Autodesk Fusion 360 part; units mm, degrees
(part 6 of 6)
sketch "Sketch1" plane through (0, 0, 0) normal (0, 0, 1) x (1, 0, 0)
  circle A0 centre (0, 0) radius 18.6 construction
  line L0 (-40.1145, 10.4906) -> (-17.9049, -15.3744)
  line L1 (5, 25.3685) -> (5, 26.9321) construction
  line L2 (-5, 26.019) -> (-5, 25.3685)
  line L3 (-5, 40) -> (-36.5447, 26.1628)
  line L4 (-28.8171, 18.6328) -> (-7.8034, 27.8505)
  line L5 (-29.888, 13.9311) -> (-26.2116, 9.6495)
  arc A1 (-36.5447, 26.1628) -> (-40.1145, 10.4906) centre (-32.5276, 17.0051) ccw
  line L6 (15.2, 40) -> (15.2, 36.8) construction
  line L7 (15.2, 36.8) -> (0, 36.8) construction
  line L8 (0, 36.8) -> (0, 40) construction
  line L9 (15.2, 40) -> (55, 40) construction
  line L10 (70.2, 40) -> (70.2, 36.8) construction
  line L11 (70.2, 36.8) -> (55, 36.8) construction
  line L12 (55, 36.8) -> (55, 40) construction
  line L13 (-5, 40) -> (0, 40) construction
  line L14 (41.6, 0) -> (41.6, 20) construction
  arc A2 (90, 30) -> (90, 40) centre (90, 35) ccw construction
  line L15 (90, 30) -> (51.6, 30) construction
  line L16 (8, 29.9321) -> (28.6, 29.9321) construction
  line L17 (31.6, 26.9321) -> (31.6, 12.775) construction
  arc A3 (-17.9049, -15.3744) -> (-13.0046, -19.6936) centre (0, 0) ccw
  arc A4 (21.5214, 9.6845) -> (7.0977, 22.5074) centre (0, 0) ccw construction
  arc A5 (-7.0977, 22.5074) -> (-21.236, 10.2952) centre (0, 0) ccw
  arc A6 (22.9714, -5.4105) -> (41.6, 0) centre (31.5, 0) ccw construction
  arc A7 (29.2641, 9.8494) -> (25.9158, 8.4159) centre (31.5, 0) ccw construction
  arc A8 (-28.8171, 18.6328) -> (-29.888, 13.9311) centre (-27.612, 15.8855) ccw
  arc A9 (-26.2116, 9.6495) -> (-21.236, 10.2952) centre (-23.9355, 11.6039) ccw
  arc A10 (-7.0977, 22.5074) -> (-5, 25.3685) centre (-8, 25.3685) ccw
  arc A11 (-5, 26.019) -> (-7.8034, 27.8505) centre (-7, 26.019) ccw
  arc A12 (8, 29.9321) -> (5, 26.9321) centre (8, 26.9321) ccw construction
  arc A13 (5, 25.3685) -> (7.0977, 22.5074) centre (8, 25.3685) ccw construction
  arc A14 (21.5214, 9.6845) -> (25.9158, 8.4159) centre (24.2571, 10.9156) ccw construction
  arc A15 (29.2641, 9.8494) -> (31.6, 12.775) centre (28.6, 12.775) ccw construction
  arc A16 (31.6, 26.9321) -> (28.6, 29.9321) centre (28.6, 26.9321) ccw construction
  arc A17 (51.6, 30) -> (41.6, 20) centre (51.6, 20) ccw construction
  line L18 (0, 40) -> (-5, 40) construction
  line L19 (90, 40) -> (70.2, 40) construction
  line L20 (55, 40) -> (15.2, 40) construction
  line L21 (-2, 36) -> (2, 36) construction
  line L22 (2, 36) -> (2, 25) construction
  line L23 (2, 25) -> (-2, 25) construction
  line L24 (-2, 25) -> (-2, 36) construction
  line L25 (-2, 33) -> (2, 33) construction
  line L26 (2, 33) -> (2, 28) construction
  line L27 (2, 28) -> (-2, 28) construction
  line L28 (-2, 28) -> (-2, 33) construction
  line L29 (34.6, 35) -> (38.6, 35) construction
  line L30 (38.6, 35) -> (38.6, 15) construction
  line L31 (38.6, 15) -> (34.6, 15) construction
  line L32 (34.6, 15) -> (34.6, 35) construction
  line L33 (34.6, 32) -> (38.6, 32) construction
  line L34 (34.6, 18) -> (38.6, 18) construction
  circle A18 centre (31.5, 0) radius 5.1 construction
  line L35 (-5, 40) -> (-36, 37) construction
  line L36 (-13.0046, -19.6936) -> (-61, 12) construction
  line L37 (-61, 12) -> (-66, 21) construction
  line L38 (-66, 21) -> (-58, 29) construction
  line L39 (-58, 29) -> (-36, 37) construction
  spline S0 degree 5 poles (-13.0046, -19.6936) (-14.6717, -18.8707) (-17.9583, -17.2189) (-22.7454, -14.7231) (-28.8419, -11.3592) (-35.9733, -7.1012) (-42.5874, -2.8108) (-48.6329, 1.4661) (-54.0317, 5.6589) (-58.666, 9.6455) (-62.3871, 13.2866) (-64.9717, 16.3085) (-66.2833, 18.8068) (-66.2897, 21.069) (-65.0586, 23.3576) (-62.7653, 25.7223) (-59.6375, 28.0847) (-55.9087, 30.3119) (-51.7598, 32.3074) (-47.3069, 34.0337) (-42.6215, 35.4885) (-37.7413, 36.6937) (-32.6835, 37.6814) (-27.4591, 38.4784) (-22.0771, 39.1028) (-16.5436, 39.5668) (-11.9988, 39.8152) (-8.5248, 39.9339) (-6.1798, 39.983) (-5, 40) knots 0 0 0 0 0 0 0.04 0.08 0.12 0.16 0.2 0.24 0.28 0.32 0.36 0.4 0.44 0.48 0.52 0.56 0.6 0.64 0.68 0.72 0.76 0.8 0.84 0.88 0.92 0.96 1 1 1 1 1 1
  line L40 (-54.565, 5.5612) -> (-67.435, 18.4389)
  line L41 (-5, 40) -> (0, 40)
  line L42 (0, 40) -> (0, 23.6)
  line L43 (0, 23.6) -> (0, 18.6)
  line L44 (-13.0046, -19.6936) -> (-10.2494, -15.5213)
  arc A19 (0, 18.6) -> (-10.2494, -15.5213) centre (0, 0) ccw
  arc A20 (-13.0046, -19.6936) -> (22.9714, -5.4105) centre (0, 0) ccw construction
  dimension "d4" = 37.2
  dimension "d6" = 47.2
  dimension "d7" = 20.2
  dimension "d8" = 20
  dimension "d11" = 31.5
  dimension "d12" = 15.2
  dimension "d13" = 3.2
  dimension "d14" = 55
  dimension "d15" = 15.2
  dimension "d16" = 3.2
  dimension "d19" = 3
  dimension "d20" = 2
  dimension "d21" = 3
  dimension "d22" = 10
  dimension "d26" = 4
  dimension "d27" = 20
  dimension "d35" = 10.2
  constraint coincident A0.centre A3.centre
  constraint coincident L0.end A4
  constraint tangent L0 A4
  constraint tangent L0 A1
  constraint parallel L0 L5
  constraint tangent L3 A1
  constraint vertical L6
  constraint horizontal L7
  constraint vertical L8
  constraint perpendicular L6 L9
  constraint vertical L10
  constraint horizontal L11
  constraint vertical L12
  constraint tangent L14 A6
  constraint perpendicular L9 L14
  constraint tangent A2 L19
  constraint tangent A2 L15
  constraint perpendicular L14 L15
  constraint concentric A3 A4
  constraint concentric A4 A5
  constraint concentric A6 A7
  constraint tangent L4 A8
  constraint tangent L5 A8
  constraint tangent L5 A9
  constraint tangent A5 A9
  constraint equal A8 A9
  constraint tangent L2 A10
  constraint tangent A5 A10
  constraint equal A8 A10
  constraint tangent L4 A11
  constraint tangent L2 A11
  constraint tangent L16 A12
  constraint tangent L1 A12
  constraint tangent L1 A13
  constraint tangent A4 A13
  constraint equal A12 A13
  constraint tangent A4 A14
  constraint tangent A7 A14
  constraint equal A12 A14
  constraint tangent L17 A15
  constraint tangent A7 A15
  constraint equal A12 A15
  constraint tangent L16 A16
  constraint tangent L17 A16
  constraint equal A12 A16
  constraint tangent L15 A17
  constraint tangent L14 A17
  constraint collinear L18 L19
  constraint collinear L19 L20
  constraint horizontal L21
  constraint vertical L22
  constraint horizontal L23
  constraint vertical L24
  constraint horizontal L25
  constraint vertical L26
  constraint horizontal L27
  constraint vertical L28
  constraint coincident L22 L26.end
  constraint coincident L24 L25.start
  constraint horizontal L29
  constraint vertical L30
  constraint horizontal L31
  constraint vertical L32
  constraint perpendicular L32 L33
  constraint perpendicular L32 L34
  constraint coincident L30 L34.end
  constraint coincident L32 L34.start
  constraint coincident L32 L33.start
  constraint coincident L30 L33.end
  constraint concentric A6 A18
  constraint tangent A3 L36
  constraint midpoint L36.end L40
  constraint perpendicular L23 L42
  constraint parallel L42 L43
  constraint coincident A0 L43.end
  constraint perpendicular L36 L44
  constraint concentric A3 A20
  measures "d4" diameter of A0
  measures "d6" diameter of A4
  measures "d7" diameter of A6
  measures "d8" diameter of A1
  measures "d11" distance of A0.centre A6.centre
  measures "d12" distance of L8.end L6.start
  measures "d13" distance of L8.end L7.end
  measures "d14" distance of L8.end L9.end
  measures "d15" distance of L9.end L10.start
  measures "d16" distance of L9.end L11.end
  measures "d19" radius of A8
  measures "d20" radius of A11
  measures "d21" radius of A12
  measures "d22" radius of A17
  measures "d26" distance of L29.start L29.end
  measures "d27" distance of L29.start L31.end
  measures "d35" diameter of A18
extrude "Extrude6" add sketch "Sketch1" along normal mid plane 16 contours L0 L3 A1 A3 L41 L42 L43 L44 A19 | L0 L3 A1 A3 S0 | L2 L4 L5 A5 A8 A9 A10 A11
extrude "Extrude7" cut sketch "Sketch1" along normal mid plane 13 contours L0 L3 A1 A3 L41 L42 L43 L44 A19 | L2 L4 L5 A5 A8 A9 A10 A11
sketch "Sketch2" plane through (0, 0, 0) normal (0, 1, 0) x (1, 0, 0)
  line L0 (-25, -15) -> (-25, 15)
  ellipse E0 centre (-25, 0) end of major axis (-66, 0) minor radius 8
  line L1 (16, 0) -> (-66, 0) construction
  line L2 (-25, 8) -> (-25, -8) construction
  line L3 (-25, -8) -> (-70, -8)
  line L4 (-70, -8) -> (-70, 8)
  line L5 (-70, 8) -> (-25, 8)
  line L6 (-25, 8) -> (-25, -8)
  constraint vertical L0
  constraint coincident E0 L1.start
  constraint coincident E0 L1.end
  constraint coincident E0 L2.start
  constraint coincident E0 L2.end
  constraint midpoint L0 E0.centre
  constraint perpendicular L0 L1
  constraint horizontal L3
  constraint vertical L4
  constraint horizontal L5
  constraint vertical L6
  constraint coincident L2.end L3.start
extrude "Extrude8" cut sketch "Sketch2" along normal mid plane 115.048 contours E0 L3 L4 L5
chamfer "Chamfer1" distance 6 distance2 1.5 6 edges at (-11.627, -17.6074, 8) (-17.8137, 5.3509, 8) (0, 29.3, 8) (0, 29.3, -8) (-17.8137, 5.3509, -8) (-11.627, -17.6074, -8) measured on face at (-12.5639, 31.8918, 8) measured on face at (-12.5639, 31.8918, 8) measured on face at (-12.5639, 31.8918, 8) measured on face at (-12.5639, 31.8918, -8) measured on face at (-12.5639, 31.8918, -8) measured on face at (-12.5639, 31.8918, -8)
fillet "Fillet1" radius 1.5 6 edges at (-15.7107, 39.5818, 8) (-61.7676, 26.3831, -3.5398) (-15.7107, 39.5818, -8) (-21.7404, -15.2089, 8) (-58.156, 9.3027, 4.706) (-21.7404, -15.2089, -8)
equation "d6 = 37.200 mm + 5 mm + 5 mm"
equation "d7 = 10.200 mm + 10 mm"

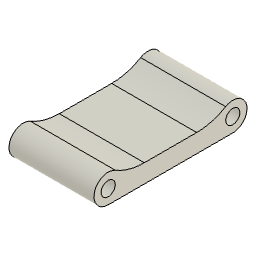
design "pivots"
Autodesk Fusion 360 part; units mm, degrees
sketch "Sketch1" plane through (0, 0, 0) normal (1, 0, 0) x (0, 1, 0)
  line L0 (0, 0) -> (17, 0)
  circle A0 centre (20, 2.5) radius 1.25
  line L1 (-2, 0) -> (20, 0)
  line L2 (13.6213, 3.25) -> (4.3787, 3.25)
  arc A1 (-0.7243, 4.65) -> (-2, 0) centre (-2, 2.5) ccw
  arc A2 (20, 0) -> (18.7243, 4.65) centre (20, 2.5) ccw
  arc A3 (-0.7243, 4.65) -> (4.3787, 3.25) centre (4.3787, 13.25) ccw
  arc A4 (13.6213, 3.25) -> (18.7243, 4.65) centre (13.6213, 13.25) ccw
  circle A5 centre (-2, 2.5) radius 1.25
  dimension "d1" = 17
  dimension "d7" = 2.5
  dimension "d8" = 10
  dimension "d11" = 2.5
  constraint horizontal L0
  constraint coincident L0.start origin
  constraint concentric A0 A2
  constraint tangent L1 A2
  constraint parallel L0 L1
  constraint tangent L2 A3
  constraint tangent A1 A3
  constraint tangent L2 A4
  constraint tangent A2 A4
  constraint equal A3 A4
  constraint concentric A1 A5
  measures "d1" distance of L0.start L0.end
  measures "d7" diameter of A0
  measures "d8" radius of A3
  measures "d11" diameter of A5
extrude "Extrude1" add sketch "Sketch1" along normal blind 20 contours L0 L1 L2 A1 A2 A3 A4 | A0 | A5
extrude "Extrude2" cut sketch "Sketch1" along normal blind 50 contours A0
extrude "Extrude3" cut sketch "Sketch1" along normal blind 25.474 contours A5
extrude "Extrude4" cut 1 faces at (20, 7.4596, 1.0833) along direction (-1, 0, 0) blind 5
equation "d1 = 2 mm + 13 mm + 2 mm"

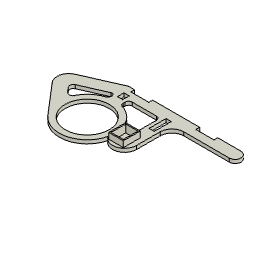
design "top_chassis"
Autodesk Fusion 360 part; units mm, degrees
sketch "Sketch1" plane through (0, 0, 0) normal (0, 0, 1) x (1, 0, 0)
  circle A0 centre (0, 0) radius 18.6
  line L0 (-40.1145, 10.4906) -> (-17.9049, -15.3744)
  line L1 (5, 25.3685) -> (5, 26.9321)
  line L2 (-5, 26.019) -> (-5, 25.3685)
  line L3 (-5, 40) -> (-36.5447, 26.1628)
  line L4 (-28.8171, 18.6328) -> (-7.8034, 27.8505)
  line L5 (-29.888, 13.9311) -> (-26.2116, 9.6495)
  arc A1 (-36.5447, 26.1628) -> (-40.1145, 10.4906) centre (-32.5276, 17.0051) ccw
  line L6 (15.2, 40) -> (15.2, 36.8)
  line L7 (15.2, 36.8) -> (0, 36.8)
  line L8 (0, 36.8) -> (0, 40)
  line L9 (15.2, 40) -> (55, 40)
  line L10 (70.2, 40) -> (70.2, 36.8)
  line L11 (70.2, 36.8) -> (55, 36.8)
  line L12 (55, 36.8) -> (55, 40)
  line L13 (-5, 40) -> (0, 40)
  line L14 (41.6, 0) -> (41.6, 20)
  arc A2 (90, 30) -> (90, 40) centre (90, 35) ccw
  line L15 (90, 30) -> (51.6, 30)
  line L16 (8, 29.9321) -> (28.6, 29.9321)
  line L17 (31.6, 26.9321) -> (31.6, 12.775)
  arc A3 (-17.9049, -15.3744) -> (22.9714, -5.4105) centre (0, 0) ccw
  arc A4 (21.5214, 9.6845) -> (7.0977, 22.5074) centre (0, 0) ccw
  arc A5 (-7.0977, 22.5074) -> (-21.236, 10.2952) centre (0, 0) ccw
  arc A6 (22.9714, -5.4105) -> (41.6, 0) centre (31.5, 0) ccw
  arc A7 (29.2641, 9.8494) -> (25.9158, 8.4159) centre (31.5, 0) ccw
  arc A8 (-28.8171, 18.6328) -> (-29.888, 13.9311) centre (-27.612, 15.8855) ccw
  arc A9 (-26.2116, 9.6495) -> (-21.236, 10.2952) centre (-23.9355, 11.6039) ccw
  arc A10 (-7.0977, 22.5074) -> (-5, 25.3685) centre (-8, 25.3685) ccw
  arc A11 (-5, 26.019) -> (-7.8034, 27.8505) centre (-7, 26.019) ccw
  arc A12 (8, 29.9321) -> (5, 26.9321) centre (8, 26.9321) ccw
  arc A13 (5, 25.3685) -> (7.0977, 22.5074) centre (8, 25.3685) ccw
  arc A14 (21.5214, 9.6845) -> (25.9158, 8.4159) centre (24.2571, 10.9156) ccw
  arc A15 (29.2641, 9.8494) -> (31.6, 12.775) centre (28.6, 12.775) ccw
  arc A16 (31.6, 26.9321) -> (28.6, 29.9321) centre (28.6, 26.9321) ccw
  arc A17 (51.6, 30) -> (41.6, 20) centre (51.6, 20) ccw
  line L18 (0, 40) -> (-5, 40)
  line L19 (90, 40) -> (70.2, 40)
  line L20 (55, 40) -> (15.2, 40)
  line L21 (34.4, 17.8) -> (38.8, 17.8)
  line L22 (38.8, 32.2) -> (38.8, 17.8)
  line L23 (34.4, 32.2) -> (38.8, 32.2)
  line L24 (34.4, 17.8) -> (34.4, 32.2)
  line L25 (2.2, 27.8) -> (-2.2, 27.8)
  line L26 (-2.2, 27.8) -> (-2.2, 33.2)
  line L27 (-2.2, 33.2) -> (2.2, 33.2)
  line L28 (2.2, 33.2) -> (2.2, 27.8)
  circle A18 centre (31.5, 0) radius 1.6
  line L29 (36.65, -6.15) -> (26.35, -6.15)
  line L30 (26.35, -6.15) -> (26.35, 6.15)
  line L31 (26.35, 6.15) -> (36.65, 6.15)
  line L32 (36.65, 6.15) -> (36.65, -6.15)
  line L33 (37.65, -7.15) -> (25.35, -7.15)
  line L34 (25.35, -7.15) -> (25.35, 7.15)
  line L35 (25.35, 7.15) -> (37.65, 7.15)
  line L36 (37.65, 7.15) -> (37.65, -7.15)
  dimension "d4" = 37.2
  dimension "d6" = 47.2
  dimension "d7" = 20.2
  dimension "d8" = 20
  dimension "d11" = 31.5
  dimension "d12" = 15.2
  dimension "d13" = 3.2
  dimension "d14" = 55
  dimension "d15" = 15.2
  dimension "d16" = 3.2
  dimension "d19" = 3
  dimension "d20" = 2
  dimension "d21" = 3
  dimension "d22" = 10
  dimension "d29" = 4.4
  dimension "d30" = 14.4
  dimension "d32" = 4.4
  dimension "d33" = 5.4
  dimension "d36" = 3.2
  constraint coincident A0.centre A3.centre
  constraint coincident L0.end A4
  constraint tangent L0 A4
  constraint tangent L0 A1
  constraint parallel L0 L5
  constraint tangent L3 A1
  constraint vertical L6
  constraint horizontal L7
  constraint vertical L8
  constraint perpendicular L6 L9
  constraint vertical L10
  constraint horizontal L11
  constraint vertical L12
  constraint tangent L14 A6
  constraint perpendicular L9 L14
  constraint tangent A2 L19
  constraint tangent A2 L15
  constraint perpendicular L14 L15
  constraint concentric A3 A4
  constraint concentric A4 A5
  constraint concentric A6 A7
  constraint tangent L4 A8
  constraint tangent L5 A8
  constraint tangent L5 A9
  constraint tangent A5 A9
  constraint equal A8 A9
  constraint tangent L2 A10
  constraint tangent A5 A10
  constraint equal A8 A10
  constraint tangent L4 A11
  constraint tangent L2 A11
  constraint tangent L16 A12
  constraint tangent L1 A12
  constraint tangent L1 A13
  constraint tangent A4 A13
  constraint equal A12 A13
  constraint tangent A4 A14
  constraint tangent A7 A14
  constraint equal A12 A14
  constraint tangent L17 A15
  constraint tangent A7 A15
  constraint equal A12 A15
  constraint tangent L16 A16
  constraint tangent L17 A16
  constraint equal A12 A16
  constraint tangent L15 A17
  constraint tangent L14 A17
  constraint collinear L18 L19
  constraint collinear L19 L20
  constraint concentric A6 A18
  measures "d4" diameter of A0
  measures "d6" diameter of A4
  measures "d7" diameter of A6
  measures "d8" diameter of A1
  measures "d11" distance of A0.centre A6.centre
  measures "d12" distance of L8.end L6.start
  measures "d13" distance of L8.end L7.end
  measures "d14" distance of L8.end L9.end
  measures "d15" distance of L9.end L10.start
  measures "d16" distance of L9.end L11.end
  measures "d19" radius of A8
  measures "d20" radius of A11
  measures "d21" radius of A12
  measures "d22" radius of A17
  measures "d29" distance of L22.start L23.start
  measures "d30" distance of L21.end L22.start
  measures "d32" distance of L26.end L27.end
  measures "d33" distance of L25.start L27.end
  measures "d36" diameter of A18
extrude "Extrude2" add sketch "Sketch1" against normal blind 3 contours L0 L3 A1 L6 L7 L8 L9 L10 L11 L12 L13 L14 A2 L15 A3 A6 A17 L18 L19 L20 | L29 L30 L31 L32 | L33 L34 L35 L36
extrude "Extrude3" cut sketch "Sketch1" against normal blind 1.5 contours L29 L30 L31 L32
extrude "Extrude4" add sketch "Sketch1" along normal blind 5 contours L33 L34 L35 L36
equation "d6 = 37.200 mm + 5 mm + 5 mm"
equation "d7 = 10.200 mm + 10 mm"

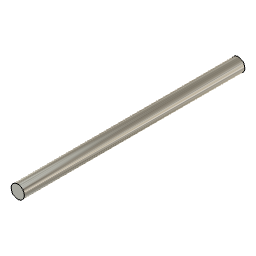
design "50mm rod"
Autodesk Fusion 360 part; units mm, degrees
sketch "Sketch1" plane through (0, 0, 0) normal (0, 1, 0) x (1, 0, 0)
  circle A0 centre (0, 0) radius 1.5
  dimension "d1" = 3
  constraint coincident A0.centre origin
  measures "d1" diameter of A0
extrude "Extrude1" add sketch "Sketch1" along normal blind 50
